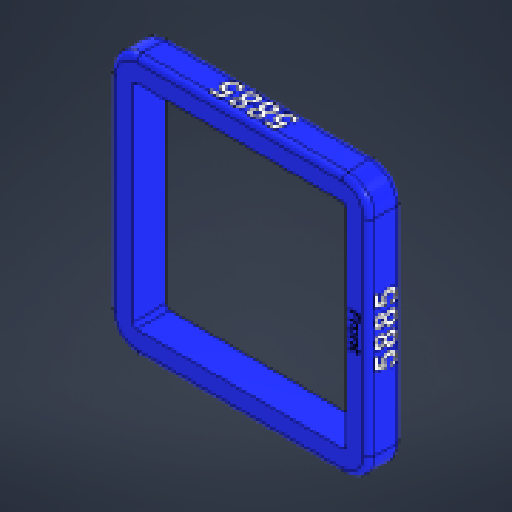
# Autodesk Inventor part: Bumpers
Saved by Autodesk Inventor 2026.1 (Build 301233020, 233B)
## iProperties
Created: 2026-01-21
Part Number: Bumpers
Material: Spruce
Document SubType Name: Modeling
Designer: Jthib
Mass: 9348.75 g
Surface Area: 10216.2 cm^2
Volume: 23371.9 cm^3
Density: 0.4 g/cm^3
Appearance: Blue - Wall Paint - Glossy
Author: Jthib
Autodesk Inventor part; units mm, degrees
ref_plane "YZ Plane" through (0, 0, 0) normal (1, 0, 0) x (0, 1, 0)
ref_plane "XZ Plane" through (0, 0, 0) normal (0, 1, 0) x (-1, 0, 0)
ref_plane "XY Plane" through (0, 0, 0) normal (0, 0, 1) x (1, 0, 0)
sketch "Sketch1" plane through (0, 0, 0) normal (0, 0, 1) x (1, 0, 0)
  line L0 (-349.25, 0) -> (-349.25, 336.55)
  line L1 (-336.55, 349.25) -> (336.55, 349.25)
  line L2 (349.25, 336.55) -> (349.25, -336.55)
  line L3 (336.55, -349.25) -> (-336.55, -349.25)
  line L4 (-349.25, -336.55) -> (-349.25, 0)
  arc A0 (-336.55, 349.25) -> (-349.25, 336.55) centre (-336.55, 336.55) ccw
  arc A1 (349.25, 336.55) -> (336.55, 349.25) centre (336.55, 336.55) ccw
  arc A2 (336.55, -349.25) -> (349.25, -336.55) centre (336.55, -336.55) ccw
  arc A3 (-349.25, -336.55) -> (-336.55, -349.25) centre (-336.55, -336.55) ccw
  point P0 (0, 0)
  point P1 (-349.25, 349.25)
  point P2 (349.25, 349.25)
  point P3 (349.25, -349.25)
  point P4 (-349.25, -349.25)
  dimension "d0" = 698.5
  dimension "d1" = 698.5
  dimension "d2" = 349.25
  dimension "d3" = 349.25
  dimension "d9" = 12.7
  constraints: 10 end point, 9 point on line, 8 point on circle, 8 tangent, 4 centre point, 4 perpendicular, 3 equal radius, 1 collinear, 1 vertical
  measures "d0" distance of point (349.25, 349.25) point (349.25, -349.25)
  measures "d1" distance of point (-349.25, 349.25) point (349.25, 349.25)
  measures "d2" distance from line of point (0, 0) L1
  measures "d3" distance from line of L2 point (0, 0)
  measures "d9" radius of A0
sketch "Sketch2" plane through (0, 0, 0) normal (0, 1, 0) x (-1, 0, 0)
  line L0 (406.4, 53.975) -> (349.25, 53.975)
  line L1 (349.25, 53.975) -> (349.25, -53.975)
  line L2 (349.25, -53.975) -> (406.4, -53.975)
  line L3 (425.45, -34.925) -> (425.45, 34.925)
  arc A0 (425.45, 34.925) -> (406.4, 53.975) centre (406.4, 34.925) ccw
  arc A1 (406.4, -53.975) -> (425.45, -34.925) centre (406.4, -34.925) ccw
  point P0 (0, 0)
  point P1 (425.45, 53.975)
  point P2 (349.25, 0)
  point P3 (349.25, 0)
  point P4 (349.25, 0)
  point P5 (349.25, 0)
  dimension "d4" = 107.95
  dimension "d5" = 76.2
  dimension "d6" = 19.05
  constraints: 8 end point, 4 point on circle, 4 tangent, 2 centre point, 2 parallel, 2 point on line, 1 coincident, 1 equal radius, 1 horizontal, 1 midpoint, 1 perpendicular
  measures "d4" distance of L0.end L1.end
  measures "d5" distance of point (425.45, 53.975) L0.end
  measures "d6" radius of A0
sweep "Sweep1" add profiles "Sketch2" path "Sketch1" path curves L0 A0 L1 A1 L2 A2 L3 A3 L4
sketch "Sketch3" plane through (425.45, -336.55, 34.925) normal (1, 0, 0) x (0, 0, -1)
  line L0 (-9.525, 82.55) -> (-9.525, 590.55) construction
  line L1 (-9.525, 590.55) -> (79.375, 590.55) construction
  line L2 (79.375, 590.55) -> (79.375, 82.55) construction
  line L3 (79.375, 82.55) -> (-9.525, 82.55) construction
  line L4 (-9.525, 82.55) -> (79.375, 590.55) construction
  line L5 (50.6645, 224.9216) -> (49.3867, 239.4995)
  spline S0 degree 2 poles (49.3867, 239.4995) (50.4322, 239.4415) (50.9549, 239.4415) knots 0 0 0 1 1 1
  spline S1 degree 2 poles (50.9549, 239.4415) (56.2401, 239.4415) (61.5253, 244.1459) (61.5253, 247.921) knots 0 0 0 1 2 2 2
  spline S2 degree 2 poles (61.5253, 247.921) (61.5253, 253.2063) (51.4195, 261.8601) (42.4753, 261.8601) knots 0 0 0 1 2 2 2
  spline S3 degree 2 poles (42.4753, 261.8601) (37.1901, 261.8601) (31.7887, 256.9814) (31.7887, 252.9159) knots 0 0 0 1 2 2 2
  spline S4 degree 2 poles (31.7887, 252.9159) (31.7887, 250.0119) (34.5184, 244.5524) (37.2482, 241.997) knots 0 0 0 1 2 2 2
  line L6 (37.2482, 241.997) -> (36.3189, 229.7422)
  line L7 (36.3189, 229.7422) -> (-2.6523, 241.3581)
  line L8 (-2.6523, 241.3581) -> (-2.6523, 279.6323)
  line L9 (-2.6523, 279.6323) -> (10.9963, 276.8445)
  line L10 (10.9963, 276.8445) -> (10.9963, 251.522)
  line L11 (10.9963, 251.522) -> (22.7284, 248.0372)
  spline S5 degree 2 poles (22.7284, 248.0372) (21.741, 250.2442) (20.7537, 254.6002) (20.7537, 256.7491) knots 0 0 0 1 2 2 2
  spline S6 degree 2 poles (20.7537, 256.7491) (20.7537, 265.461) (32.4857, 276.6703) (42.3591, 276.6703) knots 0 0 0 1 2 2 2
  spline S7 degree 2 poles (42.3591, 276.6703) (50.2579, 276.6703) (65.5909, 268.8296) (73.78, 254.8906) (73.78, 247.2822) knots 0 0 0 1 2 3 3 3
  spline S8 degree 2 poles (73.78, 247.2822) (73.78, 237.5249) (61.2349, 225.0378) (50.6645, 224.9216) knots 0 0 0 1 2 2 2
  spline S9 degree 2 poles (30.5691, 300.2505) (27.9555, 296.243) (20.986, 292.2355) (16.8043, 292.2355) knots 0 0 0 1 2 2 2
  spline S10 degree 2 poles (16.8043, 292.2355) (11.8675, 292.2355) (1.7617, 297.8692) (-4.0462, 309.0204) (-4.0462, 316.1061) knots 0 0 0 1 2 3 3 3
  spline S11 degree 2 poles (-4.0462, 316.1061) (-4.0462, 326.27) (6.5823, 337.7116) (14.7134, 337.7116) knots 0 0 0 1 2 2 2
  spline S12 degree 2 poles (14.7134, 337.7116) (20.4052, 337.7116) (28.9428, 331.2648) (31.7306, 324.818) knots 0 0 0 1 2 2 2
  spline S13 degree 2 poles (31.7306, 324.818) (34.5765, 329.4643) (42.7657, 334.1107) (47.9928, 334.1107) knots 0 0 0 1 2 2 2
  spline S14 degree 2 poles (47.9928, 334.1107) (56.6466, 334.1107) (63.7323, 328.5931) knots 0 0 0 1 1 1
  spline S15 degree 2 poles (63.7323, 328.5931) (73.8962, 320.5782) (73.8962, 306.7553) knots 0 0 0 1 1 1
  spline S16 degree 2 poles (73.8962, 306.7553) (73.8962, 296.6495) (61.9899, 284.3948) (52.8134, 284.3948) knots 0 0 0 1 2 2 2
  spline S17 degree 2 poles (52.8134, 284.3948) (45.147, 284.3948) (33.0665, 292.9325) (30.5691, 300.2505) knots 0 0 0 1 2 2 2
  spline S18 degree 2 poles (53.0457, 299.2631) (57.3436, 299.2631) (62.2223, 303.9095) (62.2223, 307.6846) knots 0 0 0 1 2 2 2
  spline S19 degree 2 poles (62.2223, 307.6846) (62.2223, 313.4345) (52.0003, 319.707) (46.0181, 319.707) knots 0 0 0 1 2 2 2
  spline S20 degree 2 poles (46.0181, 319.707) (42.1849, 319.707) (37.2482, 314.8864) (37.2482, 311.1694) knots 0 0 0 1 2 2 2
  spline S21 degree 2 poles (37.2482, 311.1694) (37.2482, 306.4649) (45.902, 299.2631) (53.0457, 299.2631) knots 0 0 0 1 2 2 2
  spline S22 degree 2 poles (17.7916, 305.8841) (21.3925, 305.8841) (25.8066, 310.2401) (25.8066, 313.7248) knots 0 0 0 1 2 2 2
  spline S23 degree 2 poles (25.8066, 313.7248) (25.8066, 317.7323) (19.7082, 323.8306) (15.6427, 323.8306) knots 0 0 0 1 2 2 2
  spline S24 degree 2 poles (15.6427, 323.8306) (11.9837, 323.8306) (7.3954, 319.3585) (7.3954, 315.8738) knots 0 0 0 1 2 2 2
  spline S25 degree 2 poles (7.3954, 315.8738) (7.3954, 311.7502) (13.4357, 305.8841) (17.7916, 305.8841) knots 0 0 0 1 2 2 2
  spline S26 degree 2 poles (30.5691, 359.4332) (27.9555, 355.4258) (20.986, 351.4183) (16.8043, 351.4183) knots 0 0 0 1 2 2 2
  spline S27 degree 2 poles (16.8043, 351.4183) (11.8675, 351.4183) (1.7617, 357.052) (-4.0462, 368.2032) (-4.0462, 375.2889) knots 0 0 0 1 2 3 3 3
  spline S28 degree 2 poles (-4.0462, 375.2889) (-4.0462, 385.4527) (6.5823, 396.8944) (14.7134, 396.8944) knots 0 0 0 1 2 2 2
  spline S29 degree 2 poles (14.7134, 396.8944) (20.4052, 396.8944) (28.9428, 390.4476) (31.7306, 384.0008) knots 0 0 0 1 2 2 2
  spline S30 degree 2 poles (31.7306, 384.0008) (34.5765, 388.6471) (42.7657, 393.2934) (47.9928, 393.2934) knots 0 0 0 1 2 2 2
  spline S31 degree 2 poles (47.9928, 393.2934) (56.6466, 393.2934) (63.7323, 387.7759) knots 0 0 0 1 1 1
  spline S32 degree 2 poles (63.7323, 387.7759) (73.8962, 379.761) (73.8962, 365.9381) knots 0 0 0 1 1 1
  spline S33 degree 2 poles (73.8962, 365.9381) (73.8962, 355.8323) (61.9899, 343.5776) (52.8134, 343.5776) knots 0 0 0 1 2 2 2
  spline S34 degree 2 poles (52.8134, 343.5776) (45.147, 343.5776) (33.0665, 352.1152) (30.5691, 359.4332) knots 0 0 0 1 2 2 2
  spline S35 degree 2 poles (53.0457, 358.4459) (57.3436, 358.4459) (62.2223, 363.0922) (62.2223, 366.8674) knots 0 0 0 1 2 2 2
  spline S36 degree 2 poles (62.2223, 366.8674) (62.2223, 372.6172) (52.0003, 378.8898) (46.0181, 378.8898) knots 0 0 0 1 2 2 2
  spline S37 degree 2 poles (46.0181, 378.8898) (42.1849, 378.8898) (37.2482, 374.0692) (37.2482, 370.3521) knots 0 0 0 1 2 2 2
  spline S38 degree 2 poles (37.2482, 370.3521) (37.2482, 365.6477) (45.902, 358.4459) (53.0457, 358.4459) knots 0 0 0 1 2 2 2
  spline S39 degree 2 poles (17.7916, 365.0669) (21.3925, 365.0669) (25.8066, 369.4229) (25.8066, 372.9076) knots 0 0 0 1 2 2 2
  spline S40 degree 2 poles (25.8066, 372.9076) (25.8066, 376.9151) (19.7082, 383.0134) (15.6427, 383.0134) knots 0 0 0 1 2 2 2
  spline S41 degree 2 poles (15.6427, 383.0134) (11.9837, 383.0134) (7.3954, 378.5413) (7.3954, 375.0566) knots 0 0 0 1 2 2 2
  spline S42 degree 2 poles (7.3954, 375.0566) (7.3954, 370.9329) (13.4357, 365.0669) (17.7916, 365.0669) knots 0 0 0 1 2 2 2
  line L12 (50.6645, 402.47) -> (49.3867, 417.0479)
  spline S43 degree 2 poles (49.3867, 417.0479) (50.4322, 416.9898) (50.9549, 416.9898) knots 0 0 0 1 1 1
  spline S44 degree 2 poles (50.9549, 416.9898) (56.2401, 416.9898) (61.5253, 421.6942) (61.5253, 425.4694) knots 0 0 0 1 2 2 2
  spline S45 degree 2 poles (61.5253, 425.4694) (61.5253, 430.7546) (51.4195, 439.4084) (42.4753, 439.4084) knots 0 0 0 1 2 2 2
  spline S46 degree 2 poles (42.4753, 439.4084) (37.1901, 439.4084) (31.7887, 434.5297) (31.7887, 430.4642) knots 0 0 0 1 2 2 2
  spline S47 degree 2 poles (31.7887, 430.4642) (31.7887, 427.5602) (34.5184, 422.1008) (37.2482, 419.5453) knots 0 0 0 1 2 2 2
  line L13 (37.2482, 419.5453) -> (36.3189, 407.2905)
  line L14 (36.3189, 407.2905) -> (-2.6523, 418.9064)
  line L15 (-2.6523, 418.9064) -> (-2.6523, 457.1806)
  line L16 (-2.6523, 457.1806) -> (10.9963, 454.3928)
  line L17 (10.9963, 454.3928) -> (10.9963, 429.0703)
  line L18 (10.9963, 429.0703) -> (22.7284, 425.5855)
  spline S48 degree 2 poles (22.7284, 425.5855) (21.741, 427.7925) (20.7537, 432.1485) (20.7537, 434.2974) knots 0 0 0 1 2 2 2
  spline S49 degree 2 poles (20.7537, 434.2974) (20.7537, 443.0093) (32.4857, 454.2186) (42.3591, 454.2186) knots 0 0 0 1 2 2 2
  spline S50 degree 2 poles (42.3591, 454.2186) (50.2579, 454.2186) (65.5909, 446.3779) (73.78, 432.4389) (73.78, 424.8305) knots 0 0 0 1 2 3 3 3
  spline S51 degree 2 poles (73.78, 424.8305) (73.78, 415.0732) (61.2349, 402.5861) (50.6645, 402.47) knots 0 0 0 1 2 2 2
  point P0 (34.925, 336.55)
  point P1 (34.925, 336.55)
  dimension "d2" = 349.25
  dimension "d10" = 508
  dimension "d11" = 88.9
  constraints: 2 end point, 1 coincident, 1 horizontal, 1 midpoint, 2 other
  measures "d10" distance of L0.start L0.end
  measures "d11" distance of L0.end L1.end
emboss "Emboss1" sketch "Sketch3" operation cut depth 0.254 direction (-1, 0, 0)
pattern_circular "Circular Pattern1" count 4 over 360 about axis through (0, 0, -10) along (0, 0, 1) of "Emboss1"
sketch "Sketch4" plane through (-336.55, -406.4, 53.975) normal (0, 0, 1) x (1, 0, 0)
  line L0 (685.8, 533.4) -> (685.8, 279.4) construction
  line L1 (685.8, 279.4) -> (742.95, 279.4) construction
  line L2 (742.95, 279.4) -> (742.95, 533.4) construction
  line L3 (742.95, 533.4) -> (685.8, 533.4) construction
  line L4 (685.8, 742.95) -> (685.8, 69.85) projected
  line L5 (742.95, 742.95) -> (742.95, 69.85) projected
  line L6 (729.3186, 440.4553) -> (729.3186, 458.1777)
  line L7 (729.3186, 458.1777) -> (718.574, 458.1777)
  line L8 (718.574, 458.1777) -> (718.574, 441.1964)
  line L9 (718.574, 441.1964) -> (714.0662, 441.1964)
  line L10 (714.0662, 441.1964) -> (714.0662, 458.1777)
  line L11 (714.0662, 458.1777) -> (695.7264, 458.1777)
  line L12 (695.7264, 458.1777) -> (695.7264, 463.2412)
  line L13 (695.7264, 463.2412) -> (733.8264, 463.2412)
  line L14 (733.8264, 463.2412) -> (733.8264, 440.4553)
  line L15 (733.8264, 440.4553) -> (729.3186, 440.4553)
  line L16 (719.1607, 421.1275) -> (719.1607, 421.3745)
  spline S0 degree 2 poles (719.1607, 421.3745) (719.315, 421.9302) (719.3768, 423.1344) (719.3768, 423.968) knots 0 0 0 1 2 2 2
  spline S1 degree 2 poles (719.3768, 423.968) (719.3768, 425.9131) (717.6786, 429.7417) (716.0114, 431.4707) knots 0 0 0 1 2 2 2
  line L17 (716.0114, 431.4707) -> (695.7264, 431.4707)
  line L18 (695.7264, 431.4707) -> (695.7264, 436.2872)
  line L19 (695.7264, 436.2872) -> (724.3168, 436.2872)
  line L20 (724.3168, 436.2872) -> (724.3168, 431.4707)
  line L21 (724.3168, 431.4707) -> (720.056, 431.4707)
  spline S2 degree 2 poles (720.056, 431.4707) (722.4026, 428.8463) (724.3168, 424.9251) (724.3168, 423.0726) knots 0 0 0 1 2 2 2
  spline S3 degree 2 poles (724.3168, 423.0726) (724.3168, 422.3316) (724.2551, 421.5906) (724.1624, 421.1275) knots 0 0 0 1 2 2 2
  line L22 (724.1624, 421.1275) -> (719.1607, 421.1275)
  spline S4 degree 2 poles (710.0216, 393.8955) (702.7968, 393.8955) (694.9236, 400.8425) (694.9236, 406.647) knots 0 0 0 1 2 2 2
  spline S5 degree 2 poles (694.9236, 406.647) (694.9236, 412.6059) (703.0438, 419.4293) (710.0216, 419.4293) knots 0 0 0 1 2 2 2
  spline S6 degree 2 poles (710.0216, 419.4293) (717.1846, 419.4293) (725.1196, 412.3898) (725.1196, 406.647) knots 0 0 0 1 2 2 2
  spline S7 degree 2 poles (725.1196, 406.647) (725.1196, 400.8425) (717.2155, 393.8955) (710.0216, 393.8955) knots 0 0 0 1 2 2 2
  spline S8 degree 2 poles (710.0216, 398.8664) (715.5791, 398.8664) (720.9823, 402.9111) (720.9823, 406.647) knots 0 0 0 1 2 2 2
  spline S9 degree 2 poles (720.9823, 406.647) (720.9823, 410.3829) (715.5791, 414.4584) (710.0216, 414.4584) knots 0 0 0 1 2 2 2
  spline S10 degree 2 poles (710.0216, 414.4584) (704.6184, 414.4584) (699.0609, 410.3829) (699.0609, 406.647) knots 0 0 0 1 2 2 2
  spline S11 degree 2 poles (699.0609, 406.647) (699.0609, 402.942) (704.5258, 398.8664) (710.0216, 398.8664) knots 0 0 0 1 2 2 2
  line L23 (695.7264, 366.5092) -> (695.7264, 371.3258)
  line L24 (695.7264, 371.3258) -> (712.0285, 371.3258)
  spline S12 degree 2 poles (712.0285, 371.3258) (714.0045, 371.3258) (717.4008, 371.6963) (718.4197, 372.252) knots 0 0 0 1 2 2 2
  spline S13 degree 2 poles (718.4197, 372.252) (719.5003, 372.8387) (720.55, 374.9382) (720.55, 376.7289) knots 0 0 0 1 2 2 2
  spline S14 degree 2 poles (720.55, 376.7289) (720.55, 378.5197) (718.6358, 382.3173) (717.092, 384.139) knots 0 0 0 1 2 2 2
  line L25 (717.092, 384.139) -> (695.7264, 384.139)
  line L26 (695.7264, 384.139) -> (695.7264, 388.9555)
  line L27 (695.7264, 388.9555) -> (724.3168, 388.9555)
  line L28 (724.3168, 388.9555) -> (724.3168, 384.139)
  line L29 (724.3168, 384.139) -> (721.1367, 384.139)
  spline S15 degree 2 poles (721.1367, 384.139) (723.0818, 381.9777) (725.1196, 377.8096) (725.1196, 375.463) knots 0 0 0 1 2 2 2
  spline S16 degree 2 poles (725.1196, 375.463) (725.1196, 371.264) (719.562, 366.5092) (714.2824, 366.5092) knots 0 0 0 1 2 2 2
  line L30 (714.2824, 366.5092) -> (695.7264, 366.5092)
  spline S17 degree 2 poles (695.1706, 351.1025) (695.1706, 355.0237) (699.6475, 359.4388) (704.4949, 359.4388) knots 0 0 0 1 2 2 2
  line L31 (704.4949, 359.4388) -> (720.3339, 359.4388)
  line L32 (720.3339, 359.4388) -> (720.3339, 362.6807)
  line L33 (720.3339, 362.6807) -> (724.3168, 362.6807)
  line L34 (724.3168, 362.6807) -> (724.3168, 359.4388)
  line L35 (724.3168, 359.4388) -> (732.5296, 359.4388)
  line L36 (732.5296, 359.4388) -> (732.5296, 354.6223)
  line L37 (732.5296, 354.6223) -> (724.3168, 354.6223)
  line L38 (724.3168, 354.6223) -> (724.3168, 345.7611)
  line L39 (724.3168, 345.7611) -> (720.3339, 345.7611)
  line L40 (720.3339, 345.7611) -> (720.3339, 354.6223)
  line L41 (720.3339, 354.6223) -> (706.7179, 354.6223)
  spline S18 degree 2 poles (706.7179, 354.6223) (704.5567, 354.6223) (702.1793, 354.4679) (701.1604, 353.943) knots 0 0 0 1 2 2 2
  spline S19 degree 2 poles (701.1604, 353.943) (700.265, 353.5108) (699.3697, 351.5656) (699.3697, 349.8984) knots 0 0 0 1 2 2 2
  spline S20 degree 2 poles (699.3697, 349.8984) (699.3697, 348.7251) (700.0798, 346.533) (700.2959, 346.039) knots 0 0 0 1 2 2 2
  line L42 (700.2959, 346.039) -> (700.2959, 345.7611)
  line L43 (700.2959, 345.7611) -> (695.9734, 345.7611)
  spline S21 degree 2 poles (695.9734, 345.7611) (695.6029, 347.1196) (695.1706, 349.8984) (695.1706, 351.1025) knots 0 0 0 1 2 2 2
  point P0 (336.55, 406.4)
  point P1 (742.95, 406.4)
  dimension "d2" = 349.25
  dimension "d17" = 254
  constraints: 2 midpoint, 1 collinear, 2 other
  measures "d17" distance between parallel lines of L1 L3
emboss "Emboss2" sketch "Sketch4" operation cut depth 2.54 direction (0, 0, -1)
equation "\"d0\" = d1"
equation "\"d2\" = 0.5 * d0"
equation "\"d3\" = 0.5 * d1"
body "Solid1"
